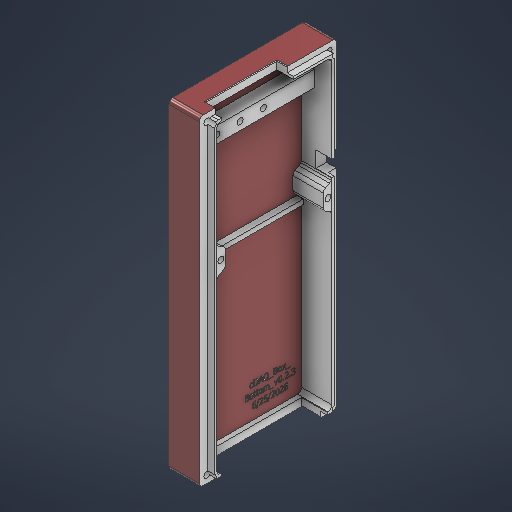
# Autodesk Inventor part: cDAQ_Box_Bottom_v0.2.3
Saved by Autodesk Inventor 2027 (Build 310192000, 192)
## iProperties
Created: 2026-05-08
Part Number: cDAQ_Box_Bottom_v0.2.3
Material: Generic
Document SubType Name: Modeling
Designer: giese
Density: 1 g/cm^3
Appearance: Default
Author: giese
Autodesk Inventor part; units mm, degrees
(part 1 of 2)
ref_plane "YZ Plane" through (0, 0, 0) normal (1, 0, 0) x (0, 1, 0)
ref_plane "XZ Plane" through (0, 0, 0) normal (0, 1, 0) x (-1, 0, 0)
ref_plane "XY Plane" through (0, 0, 0) normal (0, 0, 1) x (1, 0, 0)
sketch "Sketch1" plane through (0, 0, 0) normal (1, 0, 0) x (0, 1, 0)
  line L0 (37.5698, 60.7867) -> (-217.4462, 60.7867)
  line L1 (-217.4462, 60.7867) -> (-217.4462, -48.4333)
  line L2 (-217.4462, -48.4333) -> (37.5698, -48.4333)
  line L3 (37.5698, -48.4333) -> (37.5698, 60.7867)
  point P0 (0, 0)
  dimension "d0" = 109.22
  dimension "d1" = 255.016
  constraints: 8 end point, 2 parallel, 1 horizontal, 1 perpendicular
  measures "d0" distance of L2.end L0.start
  measures "d1" distance of L1.end L2.end
extrude "Extrusion1" add sketch "Sketch1" along normal blind 24.13
sketch "Sketch2" plane through (24.13, 0, 0) normal (1, 0, 0) x (0, 0, -1)
  line L0 (39.5433, 31.2198) -> (-51.8967, 31.2198)
  line L1 (-51.8967, 31.2198) -> (-51.8967, -211.0962)
  line L2 (-51.8967, -211.0962) -> (39.5433, -211.0962)
  line L3 (39.5433, -211.0962) -> (39.5433, 31.2198)
  line L4 (48.4333, 37.5698) -> (-60.7867, 37.5698) projected
  line L5 (-60.7867, 37.5698) -> (-60.7867, -217.4462) projected
  line L6 (-60.7867, -217.4462) -> (48.4333, -217.4462) projected
  line L7 (48.4333, -217.4462) -> (48.4333, 37.5698) projected
  point P0 (0, 0)
  dimension "d4" = 242.316
  dimension "d5" = 91.44
  dimension "d8" = 6.35
  dimension "d21" = 8.89
  dimension "d690" = 6.35
  dimension "d842" = 8.89
  constraints: 8 end point, 2 parallel, 1 horizontal, 1 perpendicular
  measures "d4" distance of L2.end L0.start
  measures "d5" distance of L0.start L0.end
  measures "d8" distance between parallel lines of L0 L4
  measures "d21" distance between parallel lines of L5 L1
  measures "d690" distance between parallel lines of L6 L2
  measures "d842" distance between parallel lines of L7 L3
extrude "Extrusion2" cut sketch "Sketch2" against normal blind 19.05 contours L3 L2 L1 L0
sketch "Sketch3" plane through (0, 0, 0) normal (-1, 0, 0) x (0, 0, 1)
  circle A0 centre (0.9291, 9.6298) radius 2.4005
  circle A1 centre (19.4279, 9.6298) radius 2.4005
  circle A2 centre (37.9267, 9.6298) radius 2.4005
  line L0 (-48.4333, -217.4462) -> (-48.4333, 37.5698) projected
  line L1 (-48.4333, 37.5698) -> (60.7867, 37.5698) projected
  line L2 (60.7867, 37.5698) -> (60.7867, -217.4462) projected
  line L3 (51.8967, 31.2198) -> (-39.5433, 31.2198) projected
  point P0 (0, 0)
  point P1 (-0.896, -23.7433)
  point P2 (-45.1848, 27.0137)
  dimension "d9" = 18.4988
  dimension "d10" = 4.801
  dimension "d11" = 4.801
  dimension "d12" = 18.4988
  dimension "d13" = 36.9976
  dimension "d18" = 22.86
  dimension "d22" = 4.801
  dimension "d58" = 27.94
  constraints: 3 centre point
  measures "d9" distance of A0.centre A1.centre
  measures "d10" diameter of A1
  measures "d11" diameter of A2
  measures "d12" distance of A1.centre A2.centre
  measures "d13" distance of A0.centre A2.centre
  measures "d18" distance from line of L2 A2.centre
  measures "d22" diameter of A0
  measures "d58" distance from line of L1 A2.centre
extrude "Extrusion3" cut sketch "Sketch3" against normal blind 5.08
sketch "Sketch5" plane through (0, -217.4462, -48.4333) normal (0, 0, -1) x (-1, 0, 0)
  line L0 (-27.2034, 165.862) -> (-16.51, 165.862)
  line L1 (-16.51, 165.862) -> (-16.51, 178.562)
  line L2 (-16.51, 178.562) -> (-27.2034, 178.562)
  line L3 (-27.2034, 178.562) -> (-27.2034, 165.862)
  line L4 (0, 255.016) -> (-24.13, 255.016) projected
  line L5 (0, 0) -> (0, 255.016) projected
  line L6 (-24.13, 0) -> (-24.13, 255.016) projected
  line L7 (0, 0) -> (-24.13, 0) projected
  point P0 (0, 217.4462)
  point P1 (-21.8567, 178.562)
  point P2 (-21.8567, 165.862)
  dimension "d28" = 10.6934
  dimension "d30" = 12.7
  dimension "d31" = 16.51
  dimension "d215" = 3.0734
  dimension "d1133" = 165.862
  constraints: 8 end point, 2 midpoint, 2 parallel, 1 horizontal, 1 perpendicular
  measures "d28" distance between parallel lines of L1 L3
  measures "d30" distance of point (-21.857, 178.562) point (-21.857, 165.862)
  measures "d31" distance between parallel lines of L5 L1
  measures "d215" distance between parallel lines of L6 L3
  measures "d1133" distance between parallel lines of L7 L0
extrude "Extrusion4" cut sketch "Sketch5" against normal blind 24.13 contours L3 L2 L6 L0 | L6 L2 L1 L0
sketch "Sketch6" plane through (0, -217.4462, -48.4333) normal (0, -1, 0) x (1, 0, 0)
  line L0 (24.08, 55.136) -> (16.08, 55.136)
  line L1 (16.08, 45.136) -> (24.08, 45.136)
  line L2 (0, 109.22) -> (0, 0) projected
  line L3 (29.63, 53.1359) -> (29.63, 47.136)
  line L4 (24.08, 55.136) -> (29.63, 53.1359)
  line L5 (29.63, 47.136) -> (24.08, 45.136)
  line L6 (0, 0) -> (24.13, 0) projected
  line L7 (24.13, 100.33) -> (24.13, 8.89) projected
  line L8 (24.13, 41.9134) -> (24.13, 37.4697)
  line L9 (16.08, 55.136) -> (8.636, 55.136)
  line L10 (8.636, 55.136) -> (8.636, 45.136)
  line L11 (8.636, 45.136) -> (21.16, 45.136)
  point P0 (0, 48.4333)
  point P1 (20.08, 55.136)
  point P2 (20.08, 45.136)
  point P3 (16.08, 50.136)
  dimension "d39" = 6
  dimension "d48" = 55.136
  dimension "d221" = 0
  dimension "d223" = 2
  dimension "d224" = 2
  dimension "d225" = 5.5
  dimension "d227" = 5.55
  dimension "d672" = 8.636
  constraints: 18 end point, 2 horizontal, 2 midpoint, 2 parallel, 2 point on line, 1 perpendicular, 1 vertical
  measures "d39" distance of L3.start L3.end
  measures "d48" distance between parallel lines of L6 L0
  measures "d221" horizontal distance of L0.start L1.end
  measures "d223" vertical distance of L3.end L1.end
  measures "d224" vertical distance of L0.start L3.start
  measures "d225" distance between parallel lines of L3 L7
  measures "d227" distance from line of L1.end L3
  measures "d672" distance between parallel lines of L2 L10
extrude "Extrusion5" [suppressed]
sketch "Sketch7" plane through (0, 37.5698, 60.7867) normal (0, 1, 0) x (1, 0, 0)
  line L0 (31.0134, 69.85) -> (16.002, 69.85)
  line L1 (16.002, 69.85) -> (16.002, 12.7)
  line L2 (16.002, 12.7) -> (31.0134, 12.7)
  line L3 (31.0134, 12.7) -> (31.0134, 69.85)
  line L4 (0, 0) -> (24.13, 0) projected
  line L5 (0, 109.22) -> (0, 0) projected
  line L6 (24.13, 109.22) -> (24.13, 0) projected
  point P0 (0, 60.7867)
  point P1 (24.13, 69.85)
  point P2 (24.13, 12.7)
  dimension "d52" = 12.7
  dimension "d55" = 16.002
  dimension "d56" = 15.0114
  dimension "d57" = 6.8834
  dimension "d1195" = 69.85
  constraints: 8 end point, 2 parallel, 1 horizontal, 1 perpendicular
  measures "d52" distance between parallel lines of L4 L2
  measures "d55" distance between parallel lines of L5 L1
  measures "d56" distance between parallel lines of L3 L1
  measures "d57" distance between parallel lines of L6 L3
  measures "d1195" distance between parallel lines of L4 L0
extrude "Extrusion6" cut sketch "Sketch7" against normal blind 7.62
fillet "Fillet1" radius 3.175 4 edges at (12.065, 37.5698, -48.4333) (12.065, 37.5698, 60.7867) (12.065, -217.4462, -48.4333) (12.065, -217.4462, 60.7867)
sketch "Sketch8" plane through (0, 0, 0) normal (-1, 0, 0) x (0, 0, 1)
  line L0 (-0.8425, 6.0992) -> (2.6881, 6.0992)
  line L1 (-0.8425, 13.1604) -> (2.6881, 13.1604)
  line L2 (-0.8425, 6.0992) -> (-2.8809, 9.6298)
  line L3 (-0.8425, 13.1604) -> (-2.8809, 9.6298)
  line L4 (2.6881, 6.0992) -> (4.7264, 9.6298)
  line L5 (2.6881, 13.1604) -> (4.7264, 9.6298)
  circle A0 centre (0.9291, 9.6298) radius 2.4005 projected
  line L6 (17.6563, 6.0992) -> (21.1869, 6.0992)
  line L7 (17.6563, 13.1604) -> (21.1869, 13.1604)
  line L8 (17.6563, 6.0992) -> (15.6179, 9.6298)
  line L9 (17.6563, 13.1604) -> (15.6179, 9.6298)
  line L10 (21.1869, 6.0992) -> (23.2253, 9.6298)
  line L11 (21.1869, 13.1604) -> (23.2253, 9.6298)
  circle A1 centre (19.4279, 9.6298) radius 2.4005 projected
  line L12 (36.1551, 6.0992) -> (34.1167, 9.6298)
  line L13 (36.1551, 13.1604) -> (34.1167, 9.6298)
  line L14 (36.1551, 6.0992) -> (39.6857, 6.0992)
  line L15 (36.1551, 13.1604) -> (39.6857, 13.1604)
  line L16 (39.6857, 6.0992) -> (41.7241, 9.6298)
  line L17 (39.6857, 13.1604) -> (41.7241, 9.6298)
  circle A2 centre (37.9267, 9.6298) radius 2.4005 projected
  point P0 (0.9228, 6.0992)
  point P1 (19.4216, 6.0992)
  point P2 (37.9204, 6.0992)
  point P3 (-2.8809, 9.6298)
  point P4 (4.7264, 9.6298)
  point P5 (23.2253, 9.6298)
  point P6 (15.6179, 9.6298)
  point P7 (41.7241, 9.6298)
  point P8 (34.1167, 9.6298)
  dimension "d60" = 7.0612
  dimension "d61" = 120
  dimension "d62" = 120
  dimension "d63" = 120
  dimension "d64" = 120
  dimension "d65" = 3.5306
  dimension "d66" = 3.5306
  dimension "d67" = 3.5306
  dimension "d68" = 3.5306
  dimension "d69" = 3.5306
  dimension "d70" = 3.5306
  dimension "d71" = 0
  dimension "d72" = 7.6074
  dimension "d73" = 3.81
  dimension "d74" = 0
  dimension "d75" = 7.0612
  dimension "d76" = 120
  dimension "d77" = 120
  dimension "d78" = 120
  dimension "d79" = 120
  dimension "d80" = 3.5306
  dimension "d81" = 3.5306
  dimension "d82" = 3.5306
  dimension "d83" = 3.5306
  dimension "d84" = 3.5306
  dimension "d85" = 3.5306
  dimension "d86" = 0
  dimension "d87" = 7.6074
  dimension "d91" = 0
  dimension "d92" = 3.81
  dimension "d93" = 7.0612
  dimension "d94" = 120
  dimension "d95" = 120
  dimension "d96" = 120
  dimension "d97" = 120
  dimension "d98" = 3.5306
  dimension "d99" = 3.5306
  dimension "d100" = 3.5306
  dimension "d101" = 3.5306
  dimension "d102" = 3.5306
  dimension "d103" = 3.5306
  dimension "d104" = 0
  dimension "d105" = 7.6074
  dimension "d108" = 0
  dimension "d109" = 3.81
  constraints: 36 end point, 6 horizontal, 3 midpoint
  measures "d60" distance from line of point (0.923, 6.099) L1
  measures "d61" angle of L0 L2
  measures "d62" angle of L1 L3
  measures "d63" angle of L4 L0
  measures "d64" angle of L5 L1
  measures "d65" distance of L0.start L0.end
  measures "d66" distance of L1.start L1.end
  measures "d67" vertical distance of L1.start L3.end
  measures "d68" vertical distance of L0.start L2.end
  measures "d69" vertical distance of L1.end L5.end
  measures "d70" vertical distance of L0.end L4.end
  measures "d71" horizontal distance of L0.start L1.start
  measures "d72" distance of L4.end L2.end
  measures "d73" distance of A0.centre L2.end
  measures "d74" vertical distance of A0.centre L4.end
  measures "d75" distance from line of point (19.422, 6.099) L7
  measures "d76" angle of L6 L8
  measures "d77" angle of L7 L9
  measures "d78" angle of L10 L6
  measures "d79" angle of L11 L7
  measures "d80" distance of L8.start L6.end
  measures "d81" distance of L9.start L7.end
  measures "d82" vertical distance of L9.start L9.end
  measures "d83" vertical distance of L8.start L8.end
  measures "d84" vertical distance of L7.end L11.end
  measures "d85" vertical distance of L6.end L10.end
  measures "d86" horizontal distance of L8.start L9.start
  measures "d87" distance of L10.end L8.end
  measures "d91" vertical distance of A1.centre L8.end
  measures "d92" distance of A1.centre L8.end
  measures "d93" distance from line of point (37.92, 6.099) L15
  measures "d94" angle of L14 L12
  measures "d95" angle of L15 L13
  measures "d96" angle of L16 L14
  measures "d97" angle of L17 L15
  measures "d98" distance of L12.start L16.start
  measures "d99" distance of L15.start L15.end
  measures "d100" vertical distance of L15.start L13.end
  measures "d101" vertical distance of L12.start L12.end
  measures "d102" vertical distance of L15.end L17.end
  measures "d103" vertical distance of L16.start L16.end
  measures "d104" horizontal distance of L12.start L15.start
  measures "d105" distance of L16.end L12.end
  measures "d108" vertical distance of A2.centre L12.end
  measures "d109" distance of A2.centre L12.end
extrude "Extrusion7" cut sketch "Sketch8" against normal blind 5 contours L2 L3 L1 L5 L4 L0 | A0 | L8 L9 L7 L11 L10 L6 | A1 | L12 L13 L15 L17 L16 L14 | A2
sketch "Sketch9" plane through (5.08, 0, 0) normal (1, 0, 0) x (0, 0, -1)
  arc A0 (22.2689, -180.8044) -> (16.8127, -180.8044) centre (19.5408, -178.3302) ccw
  line L0 (45.2583, 37.5698) -> (9.0633, 37.5698) projected
  line L1 (39.5433, 31.2198) -> (39.5433, -38.8842) projected
  arc A1 (17.6358, -185.9502) -> (21.4458, -185.9502) centre (19.5408, -185.9502) ccw
  line L2 (21.4458, -185.9502) -> (21.4458, -182.9374)
  line L3 (17.6358, -185.9502) -> (17.6358, -182.9374)
  arc A2 (22.2689, -180.8044) -> (21.4458, -182.9374) centre (24.6208, -182.9374) ccw
  arc A3 (17.6358, -182.9374) -> (16.8127, -180.8044) centre (14.4608, -182.9374) ccw
  arc A4 (-28.5311, -180.8044) -> (-33.9873, -180.8045) centre (-31.2592, -178.3302) ccw
  arc A5 (-33.1642, -185.9366) -> (-29.3542, -185.9502) centre (-31.2592, -185.9502) ccw
  line L4 (-29.3542, -185.9502) -> (-29.3542, -182.9374)
  line L5 (-33.1642, -185.9366) -> (-33.1642, -182.9374)
  arc A6 (-28.5311, -180.8044) -> (-29.3542, -182.9374) centre (-26.1792, -182.9374) ccw
  arc A7 (-33.1642, -182.9374) -> (-33.9873, -180.8045) centre (-36.3392, -182.9374) ccw
  line L6 (-48.0867, 37.5698) -> (-57.6117, 37.5698) projected
  line L7 (-51.8967, -211.0962) -> (-51.8967, 31.2198) projected
  point P0 (0, 0)
  point P1 (39.5433, -211.0962)
  point P2 (21.4458, -181.4823)
  point P3 (17.6358, -181.4823)
  point P4 (-29.3542, -181.4823)
  point P5 (-33.1642, -181.4823)
  point P6 (-51.8967, 31.2198)
  point P7 (-49.3567, -207.2862)
  dimension "d112" = 215.9
  dimension "d114" = 7.366
  dimension "d116" = 3.81
  dimension "d117" = 223.52
  dimension "d118" = 3.175
  dimension "d119" = 7.366
  dimension "d120" = 3.81
  dimension "d121" = 3.175
  dimension "d122" = 215.9
  dimension "d123" = 223.52
  dimension "d125" = 0
  dimension "d128" = 50.8
  dimension "d129" = 20.0025
  dimension "d130" = 0
  constraints: 20 point on circle, 8 centre point, 8 end point, 8 tangent, 4 point on line, 2 equal radius, 2 parallel, 2 vertical, 1 other
  measures "d112" distance from line of L0 A0.centre
  measures "d114" diameter of A0
  measures "d116" diameter of A1
  measures "d117" distance from line of L0 A1.centre
  measures "d118" radius of A2
  measures "d119" diameter of A4
  measures "d120" diameter of A5
  measures "d121" radius of A6
  measures "d122" distance from line of A4.centre L6
  measures "d123" distance from line of L6 A5.centre
  measures "d125" horizontal distance of A5.centre A4.centre
  measures "d128" distance of A5.centre A1.centre
  measures "d129" distance from line of L1 A0.centre
  measures "d130" horizontal distance of A0.centre A1.centre
extrude "Extrusion8" [suppressed]
sketch "Sketch10" plane through (24.13, 0, 0) normal (1, 0, 0) x (0, 0, -1)
  line L0 (-51.8967, 31.2198) -> (39.5433, 31.2198) projected
  line L1 (-51.8967, 31.2198) -> (39.5433, 31.2198)
  line L2 (42.0833, 33.2264) -> (-46.8167, 33.2264)
  line L3 (-46.8167, 33.2264) -> (-53.9033, 33.2264)
  line L4 (-53.9033, 33.2264) -> (-53.9033, -213.1028)
  line L5 (-53.9033, -213.1028) -> (41.5499, -213.1028)
  line L6 (41.5499, -213.1028) -> (41.5499, 33.2264)
  line L7 (41.5499, 33.2264) -> (41.9392, 33.2264)
  line L8 (39.5433, 31.2198) -> (39.5433, -38.8842) projected
  line L9 (-51.8967, -211.0962) -> (-51.8967, 31.2198) projected
  line L10 (39.5433, -211.0962) -> (-51.8967, -211.0962) projected
  line L11 (45.2583, 37.5698) -> (9.0633, 37.5698) projected
  line L12 (39.5433, 31.2198) -> (39.5433, -211.0962)
  line L13 (39.5433, -211.0962) -> (-51.8967, -211.0962)
  line L14 (-57.6117, -217.4462) -> (45.2583, -217.4462) projected
  line L15 (-51.8967, -211.0962) -> (-51.8967, 31.2198)
  line L16 (-51.8967, 31.2198) -> (39.5433, 31.2198)
  line L17 (-51.8967, 31.2198) -> (39.5433, 31.2198)
  line L18 (39.5433, 31.2198) -> (39.5433, -211.0962)
  line L19 (39.5433, -211.0962) -> (-51.8967, -211.0962)
  line L20 (-51.8967, -211.0962) -> (-51.8967, 31.2198)
  point P0 (41.5499, 33.2264)
  point P1 (-49.3567, -207.2862)
  point P2 (39.5433, -38.8842)
  dimension "d202" = 2.0066
  dimension "d203" = 2.0066
  dimension "d204" = 2.0066
  dimension "d205" = 2.0066
  dimension "d208" = 4.3434
  constraints: 30 end point, 6 perpendicular, 3 collinear, 3 point on line, 2 horizontal, 2 parallel, 2 other
  measures "d202" distance between parallel lines of L0 L2
  measures "d203" distance between parallel lines of L6 L8
  measures "d205" distance between parallel lines of L5 L10
  measures "d208" distance between parallel lines of L11 L2
extrude "Extrusion9" add sketch "Sketch10" along normal blind 5
fillet "Fillet2" radius 3.175 7 edges at (17.105, 31.2198, -39.5433) (17.105, 31.2198, 51.8967) (17.105, -211.0962, 51.8967) (17.105, -211.0962, -39.5433) (26.63, 33.2264, 53.9033) (26.63, -213.1028, -41.5499) (26.63, -213.1028, 53.9033)
sketch "Sketch13" plane through (29.13, 0, 0) normal (1, 0, 0) x (0, 0, -1)
  arc A0 (44.0833, 30.0448) -> (40.9083, 33.2198) centre (40.9083, 30.0448) ccw projected
  arc A1 (-45.6417, 33.2198) -> (-48.8167, 30.0448) centre (-45.6417, 30.0448) ccw projected
  arc A2 (40.9083, -212.0802) -> (44.0833, -208.9052) centre (40.9083, -208.9052) ccw projected
  arc A3 (-48.8167, -208.9052) -> (-45.6417, -212.0802) centre (-45.6417, -208.9052) ccw projected
  line L0 (-48.0867, 37.5698) -> (-57.6117, 37.5698) projected
  line L1 (-60.7867, 34.3948) -> (-60.7867, -214.2712) projected
  line L2 (-57.6117, -217.4462) -> (45.2583, -217.4462) projected
  arc A4 (-48.8167, -208.9052) -> (-45.6417, -212.0802) centre (-45.6417, -208.9052) ccw projected
  circle A5 centre (-54.6907, -211.3502) radius 2.4005
  circle A6 centre (42.3373, -211.3502) radius 2.4005
  line L3 (48.4333, -214.2712) -> (48.4333, 34.3948) projected
  circle A7 centre (42.3373, 31.4738) radius 2.4005
  line L4 (45.2583, 37.5698) -> (9.0633, 37.5698) projected
  circle A8 centre (-54.6907, 31.4738) radius 2.4005
  arc A9 (41.4904, -28.6131) -> (38.3154, -25.4381) centre (38.3154, -28.6131) ccw
  circle A10 centre (36.3683, -64.0302) radius 2.4005
  circle A11 centre (-48.7217, -64.0302) radius 2.4005
  point P0 (0, 0)
  point P1 (-47.8868, 32.2898)
  point P2 (-47.8868, -211.1503)
  point P3 (-47.8868, -211.1503)
  point P4 (45.8404, -24.2631)
  point P5 (42.6654, -21.0881)
  dimension "d178" = 6.096
  dimension "d179" = 6.096
  dimension "d180" = 4.801
  dimension "d181" = 6.096
  dimension "d182" = 6.096
  dimension "d183" = 4.801
  dimension "d184" = 4.801
  dimension "d185" = 6.096
  dimension "d186" = 6.096
  dimension "d187" = 4.801
  dimension "d188" = 6.096
  dimension "d189" = 6.096
  dimension "d326" = 4.801
  dimension "d327" = 12.065
  dimension "d328" = 101.6
  dimension "d329" = 4.801
  dimension "d330" = 12.065
  dimension "d331" = 101.6
  constraints: 7 centre point, 5 point on circle
  measures "d178" distance from line of L1 A5.centre
  measures "d179" distance from line of L2 A5.centre
  measures "d180" diameter of A5
  measures "d181" distance from line of L2 A6.centre
  measures "d182" distance from line of L3 A6.centre
  measures "d183" diameter of A6
  measures "d184" diameter of A7
  measures "d185" distance from line of L3 A7.centre
  measures "d186" distance from line of L4 A7.centre
  measures "d187" diameter of A8
  measures "d188" distance from line of L0 A8.centre
  measures "d189" distance from line of L1 A8.centre
  measures "d326" diameter of A10
  measures "d327" distance from line of L3 A10.centre
  measures "d328" distance from line of A10.centre L4
  measures "d329" diameter of A11
  measures "d330" distance from line of L1 A11.centre
  measures "d331" distance from line of L0 A11.centre
extrude "Extrusion11" cut sketch "Sketch13" against normal blind 25.4
sketch "Sketch14" plane through (5.08, 0, 0) normal (1, 0, 0) x (0, 0, -1)
  line L0 (4.9426, -183.8597) -> (24.1593, -183.8597) construction
  line L1 (24.1593, -183.8597) -> (24.1593, -181.9103) construction
  line L2 (24.1593, -181.9103) -> (4.9426, -181.9103) construction
  line L3 (4.9426, -181.9103) -> (4.9426, -183.8597) construction
  spline S0 degree 2 poles (0.0458, -188.6059) (-0.3099, -188.6059) (-0.899, -188.3873) (-1.1102, -188.165) knots 0 0 0 1 2 2 2
  spline S1 degree 2 poles (-1.1102, -188.165) (-1.3214, -187.9464) (-1.5548, -187.2721) (-1.5548, -186.82) knots 0 0 0 1 2 2 2
  spline S2 degree 2 poles (-1.5548, -186.82) (-1.5548, -186.368) (-1.314, -185.7085) (-1.1102, -185.4862) knots 0 0 0 1 2 2 2
  spline S3 degree 2 poles (-1.1102, -185.4862) (-0.9064, -185.2602) (-0.3025, -185.0194) (0.0458, -185.0194) knots 0 0 0 1 2 2 2
  spline S4 degree 2 poles (0.0458, -185.0194) (0.3273, -185.0194) (0.8535, -185.1787) (1.0572, -185.2825) knots 0 0 0 1 2 2 2
  line L4 (1.0572, -185.2825) -> (1.0572, -185.9308)
  line L5 (1.0572, -185.9308) -> (1.0239, -185.9308)
  spline S5 degree 2 poles (1.0239, -185.9308) (0.9609, -185.879) (0.7682, -185.7456) (0.6312, -185.6752) knots 0 0 0 1 2 2 2
  spline S6 degree 2 poles (0.6312, -185.6752) (0.5089, -185.6159) (0.1829, -185.5233) (0.0347, -185.5233) knots 0 0 0 1 2 2 2
  spline S7 degree 2 poles (0.0347, -185.5233) (-0.4137, -185.5233) (-0.9583, -186.2013) (-0.9583, -186.82) knots 0 0 0 1 2 2 2
  spline S8 degree 2 poles (-0.9583, -186.82) (-0.9583, -187.424) (-0.4322, -188.102) (0.0347, -188.102) knots 0 0 0 1 2 2 2
  spline S9 degree 2 poles (0.0347, -188.102) (0.3162, -188.102) (0.8275, -187.8686) (1.0239, -187.687) knots 0 0 0 1 2 2 2
  line L6 (1.0239, -187.687) -> (1.0572, -187.687)
  line L7 (1.0572, -187.687) -> (1.0572, -188.3354)
  spline S10 degree 2 poles (1.0572, -188.3354) (0.972, -188.3762) (0.7127, -188.491) (0.6089, -188.5169) knots 0 0 0 1 2 2 2
  spline S11 degree 2 poles (0.6089, -188.5169) (0.4607, -188.5614) (0.2273, -188.6059) (0.0458, -188.6059) knots 0 0 0 1 2 2 2
  spline S12 degree 2 poles (5.2328, -186.2458) (5.2328, -186.8719) (4.7252, -187.8797) (4.2991, -188.1613) knots 0 0 0 1 2 2 2
  spline S13 degree 2 poles (4.2991, -188.1613) (3.9509, -188.3799) (3.2358, -188.5281) (2.68, -188.5281) knots 0 0 0 1 2 2 2
  line L8 (2.68, -188.5281) -> (1.6278, -188.5281)
  line L9 (1.6278, -188.5281) -> (1.6278, -183.9561)
  line L10 (1.6278, -183.9561) -> (2.6689, -183.9561)
  spline S14 degree 2 poles (2.6689, -183.9561) (3.3136, -183.9561) (4.0472, -184.1487) (4.3065, -184.3191) knots 0 0 0 1 2 2 2
  spline S15 degree 2 poles (4.3065, -184.3191) (4.7474, -184.6118) (5.2328, -185.5789) (5.2328, -186.2458) knots 0 0 0 1 2 2 2
  spline S16 degree 2 poles (4.5992, -186.2384) (4.5992, -185.7122) (4.251, -184.9675) (3.9064, -184.7563) knots 0 0 0 1 2 2 2
  spline S17 degree 2 poles (3.9064, -184.7563) (3.6619, -184.6118) (3.1098, -184.4822) (2.6986, -184.4822) knots 0 0 0 1 2 2 2
  line L11 (2.6986, -184.4822) -> (2.2354, -184.4822)
  line L12 (2.2354, -184.4822) -> (2.2354, -188.0019)
  line L13 (2.2354, -188.0019) -> (2.6986, -188.0019)
  spline S18 degree 2 poles (2.6986, -188.0019) (3.1024, -188.0019) (3.7137, -187.8723) (3.962, -187.6981) knots 0 0 0 1 2 2 2
  spline S19 degree 2 poles (3.962, -187.6981) (4.2806, -187.4832) (4.5992, -186.7719) (4.5992, -186.2384) knots 0 0 0 1 2 2 2
  line L14 (5.3995, -188.5281) -> (6.9408, -183.9561)
  line L15 (6.9408, -183.9561) -> (7.6892, -183.9561)
  line L16 (7.6892, -183.9561) -> (9.2305, -188.5281)
  line L17 (9.2305, -188.5281) -> (8.5896, -188.5281)
  line L18 (8.5896, -188.5281) -> (8.1746, -187.2498)
  line L19 (8.1746, -187.2498) -> (6.4295, -187.2498)
  line L20 (6.4295, -187.2498) -> (6.0146, -188.5281)
  line L21 (6.0146, -188.5281) -> (5.3995, -188.5281)
  line L22 (8.0079, -186.7311) -> (7.3002, -184.5785)
  line L23 (7.3002, -184.5785) -> (6.5962, -186.7311)
  line L24 (6.5962, -186.7311) -> (8.0079, -186.7311)
  spline S20 degree 2 poles (13.4617, -189.647) (13.2949, -189.6877) (12.9318, -189.7322) (12.7503, -189.7322) knots 0 0 0 1 2 2 2
  spline S21 degree 2 poles (12.7503, -189.7322) (12.2353, -189.7322) (11.5943, -189.1579) (11.5647, -188.6244) knots 0 0 0 1 2 2 2
  spline S22 degree 2 poles (11.5647, -188.6244) (11.5239, -188.6244) (11.4535, -188.6244) (11.4239, -188.6244) knots 0 0 0 1 2 2 2
  spline S23 degree 2 poles (11.4239, -188.6244) (10.9608, -188.6244) (10.2161, -188.3095) (9.9493, -188.0019) knots 0 0 0 1 2 2 2
  spline S24 degree 2 poles (9.9493, -188.0019) (9.6862, -187.6981) (9.4047, -186.8089) (9.4047, -186.2458) knots 0 0 0 1 2 2 2
  spline S25 degree 2 poles (9.4047, -186.2458) (9.4047, -185.6678) (9.6899, -184.7934) (9.953, -184.4822) knots 0 0 0 1 2 2 2
  spline S26 degree 2 poles (9.953, -184.4822) (10.2198, -184.1747) (10.9645, -183.8597) (11.4239, -183.8597) knots 0 0 0 1 2 2 2
  spline S27 degree 2 poles (11.4239, -183.8597) (11.8907, -183.8597) (12.6391, -184.1858) (12.8985, -184.4822) knots 0 0 0 1 2 2 2
  spline S28 degree 2 poles (12.8985, -184.4822) (13.1578, -184.7823) (13.4468, -185.6752) (13.4468, -186.2458) knots 0 0 0 1 2 2 2
  spline S29 degree 2 poles (13.4468, -186.2458) (13.4468, -187.135) (12.754, -188.2909) (12.1501, -188.4947) knots 0 0 0 1 2 2 2
  spline S30 degree 2 poles (12.1501, -188.4947) (12.1649, -188.6651) (12.2538, -188.9393) (12.3242, -189.0171) knots 0 0 0 1 2 2 2
  spline S31 degree 2 poles (12.3242, -189.0171) (12.4094, -189.1135) (12.6428, -189.2024) (12.8503, -189.2024) knots 0 0 0 1 2 2 2
  spline S32 degree 2 poles (12.8503, -189.2024) (12.9726, -189.2024) (13.306, -189.1246) (13.3801, -189.0949) knots 0 0 0 1 2 2 2
  line L25 (13.3801, -189.0949) -> (13.4617, -189.0949)
  line L26 (13.4617, -189.0949) -> (13.4617, -189.647)
  spline S33 degree 2 poles (12.8133, -186.2458) (12.8133, -185.79) (12.6169, -185.0898) (12.4391, -184.8601) knots 0 0 0 1 2 2 2
  spline S34 degree 2 poles (12.4391, -184.8601) (12.2575, -184.623) (11.7462, -184.3858) (11.4276, -184.3858) knots 0 0 0 1 2 2 2
  spline S35 degree 2 poles (11.4276, -184.3858) (11.0979, -184.3858) (10.6014, -184.6156) (10.4124, -184.8601) knots 0 0 0 1 2 2 2
  spline S36 degree 2 poles (10.4124, -184.8601) (10.2309, -185.0935) (10.0382, -185.8012) (10.0382, -186.2458) knots 0 0 0 1 2 2 2
  spline S37 degree 2 poles (10.0382, -186.2458) (10.0382, -187.1461) (10.794, -188.1057) (11.4276, -188.1057) knots 0 0 0 1 2 2 2
  spline S38 degree 2 poles (11.4276, -188.1057) (12.0612, -188.1057) (12.8133, -187.1461) (12.8133, -186.2458) knots 0 0 0 1 2 2 2
  line L27 (17.1296, -189.4469) -> (13.6024, -189.4469)
  line L28 (13.6024, -189.4469) -> (13.6024, -189.0505)
  line L29 (13.6024, -189.0505) -> (17.1296, -189.0505)
  line L30 (17.1296, -189.0505) -> (17.1296, -189.4469)
  spline S39 degree 2 poles (20.6457, -187.1239) (20.6457, -187.4647) (20.3863, -187.9871) (20.1715, -188.1576) knots 0 0 0 1 2 2 2
  spline S40 degree 2 poles (20.1715, -188.1576) (19.9121, -188.3576) (19.323, -188.5281) (18.8562, -188.5281) knots 0 0 0 1 2 2 2
  line L31 (18.8562, -188.5281) -> (17.5446, -188.5281)
  line L32 (17.5446, -188.5281) -> (17.5446, -183.9561)
  line L33 (17.5446, -183.9561) -> (18.7561, -183.9561)
  spline S41 degree 2 poles (18.7561, -183.9561) (19.2452, -183.9561) (19.7343, -184.019) (19.9566, -184.1413) knots 0 0 0 1 2 2 2
  spline S42 degree 2 poles (19.9566, -184.1413) (20.2048, -184.271) (20.4308, -184.6971) (20.4308, -184.9861) knots 0 0 0 1 2 2 2
  spline S43 degree 2 poles (20.4308, -184.9861) (20.4308, -185.3084) (20.0899, -185.8197) (19.7898, -185.9642) knots 0 0 0 1 2 2 2
  line L34 (19.7898, -185.9642) -> (19.7898, -185.9864)
  spline S44 degree 2 poles (19.7898, -185.9864) (20.1974, -186.0976) (20.6457, -186.6867) (20.6457, -187.1239) knots 0 0 0 1 2 2 2
  spline S45 degree 2 poles (20.0121, -187.1498) (20.0121, -186.8904) (19.8639, -186.557) (19.6416, -186.4384) knots 0 0 0 1 2 2 2
  spline S46 degree 2 poles (19.6416, -186.4384) (19.4971, -186.3643) (19.1563, -186.3199) (18.8414, -186.3199) knots 0 0 0 1 2 2 2
  line L35 (18.8414, -186.3199) -> (18.1522, -186.3199)
  line L36 (18.1522, -186.3199) -> (18.1522, -188.0094)
  line L37 (18.1522, -188.0094) -> (18.645, -188.0094)
  spline S47 degree 2 poles (18.645, -188.0094) (19.0451, -188.0094) (19.5046, -187.9353) (19.6824, -187.8167) knots 0 0 0 1 2 2 2
  spline S48 degree 2 poles (19.6824, -187.8167) (19.8528, -187.6944) (20.0121, -187.3906) (20.0121, -187.1498) knots 0 0 0 1 2 2 2
  spline S49 degree 2 poles (19.7973, -185.0713) (19.7973, -184.9082) (19.6861, -184.6637) (19.5638, -184.5933) knots 0 0 0 1 2 2 2
  spline S50 degree 2 poles (19.5638, -184.5933) (19.4156, -184.5118) (19.0562, -184.4748) (18.7339, -184.4748) knots 0 0 0 1 2 2 2
  line L38 (18.7339, -184.4748) -> (18.1522, -184.4748)
  line L39 (18.1522, -184.4748) -> (18.1522, -185.8123)
  line L40 (18.1522, -185.8123) -> (18.8414, -185.8123)
  spline S51 degree 2 poles (18.8414, -185.8123) (19.1266, -185.8123) (19.3971, -185.753) (19.5416, -185.6604) knots 0 0 0 1 2 2 2
  spline S52 degree 2 poles (19.5416, -185.6604) (19.6824, -185.5714) (19.7973, -185.2862) (19.7973, -185.0713) knots 0 0 0 1 2 2 2
  spline S53 degree 2 poles (24.0247, -186.8126) (24.0247, -187.6796) (23.1911, -188.6244) (22.4945, -188.6244) knots 0 0 0 1 2 2 2
  spline S54 degree 2 poles (22.4945, -188.6244) (21.7794, -188.6244) (20.9606, -187.65) (20.9606, -186.8126) knots 0 0 0 1 2 2 2
  spline S55 degree 2 poles (20.9606, -186.8126) (20.9606, -185.9531) (21.8054, -185.0009) (22.4945, -185.0009) knots 0 0 0 1 2 2 2
  spline S56 degree 2 poles (22.4945, -185.0009) (23.1911, -185.0009) (24.0247, -185.9494) (24.0247, -186.8126) knots 0 0 0 1 2 2 2
  spline S57 degree 2 poles (23.4282, -186.8126) (23.4282, -186.1457) (22.9428, -185.4973) (22.4945, -185.4973) knots 0 0 0 1 2 2 2
  spline S58 degree 2 poles (22.4945, -185.4973) (22.0462, -185.4973) (21.5571, -186.1457) (21.5571, -186.8126) knots 0 0 0 1 2 2 2
  spline S59 degree 2 poles (21.5571, -186.8126) (21.5571, -187.461) (22.0462, -188.1279) (22.4945, -188.1279) knots 0 0 0 1 2 2 2
  spline S60 degree 2 poles (22.4945, -188.1279) (22.9391, -188.1279) (23.4282, -187.4721) (23.4282, -186.8126) knots 0 0 0 1 2 2 2
  line L41 (27.2814, -188.5281) -> (26.5737, -188.5281)
  line L42 (26.5737, -188.5281) -> (25.7401, -187.2387)
  line L43 (25.7401, -187.2387) -> (24.8842, -188.5281)
  line L44 (24.8842, -188.5281) -> (24.2285, -188.5281)
  line L45 (24.2285, -188.5281) -> (25.4178, -186.8275)
  line L46 (25.4178, -186.8275) -> (24.2396, -185.0972)
  line L47 (24.2396, -185.0972) -> (24.9472, -185.0972)
  line L48 (24.9472, -185.0972) -> (25.7772, -186.3754)
  line L49 (25.7772, -186.3754) -> (26.6256, -185.0972)
  line L50 (26.6256, -185.0972) -> (27.2814, -185.0972)
  line L51 (27.2814, -185.0972) -> (26.0995, -186.7904)
  line L52 (26.0995, -186.7904) -> (27.2814, -188.5281)
  line L53 (30.7901, -189.4469) -> (27.2629, -189.4469)
  line L54 (27.2629, -189.4469) -> (27.2629, -189.0505)
  line L55 (27.2629, -189.0505) -> (30.7901, -189.0505)
  line L56 (30.7901, -189.0505) -> (30.7901, -189.4469)
  spline S61 degree 2 poles (-2.2254, -194.6515) (-2.2254, -194.9924) (-2.4848, -195.5148) (-2.6997, -195.6852) knots 0 0 0 1 2 2 2
  spline S62 degree 2 poles (-2.6997, -195.6852) (-2.959, -195.8853) (-3.5481, -196.0557) (-4.0149, -196.0557) knots 0 0 0 1 2 2 2
  line L57 (-4.0149, -196.0557) -> (-5.3265, -196.0557)
  line L58 (-5.3265, -196.0557) -> (-5.3265, -191.4837)
  line L59 (-5.3265, -191.4837) -> (-4.115, -191.4837)
  spline S63 degree 2 poles (-4.115, -191.4837) (-3.6259, -191.4837) (-3.1369, -191.5467) (-2.9145, -191.669) knots 0 0 0 1 2 2 2
  spline S64 degree 2 poles (-2.9145, -191.669) (-2.6663, -191.7987) (-2.4403, -192.2247) (-2.4403, -192.5137) knots 0 0 0 1 2 2 2
  spline S65 degree 2 poles (-2.4403, -192.5137) (-2.4403, -192.8361) (-2.7812, -193.3474) (-3.0813, -193.4919) knots 0 0 0 1 2 2 2
  line L60 (-3.0813, -193.4919) -> (-3.0813, -193.5141)
  spline S66 degree 2 poles (-3.0813, -193.5141) (-2.6737, -193.6252) (-2.2254, -194.2143) (-2.2254, -194.6515) knots 0 0 0 1 2 2 2
  spline S67 degree 2 poles (-2.859, -194.6775) (-2.859, -194.4181) (-3.0072, -194.0847) (-3.2295, -193.9661) knots 0 0 0 1 2 2 2
  spline S68 degree 2 poles (-3.2295, -193.9661) (-3.374, -193.892) (-3.7148, -193.8475) (-4.0298, -193.8475) knots 0 0 0 1 2 2 2
  line L61 (-4.0298, -193.8475) -> (-4.7189, -193.8475)
  line L62 (-4.7189, -193.8475) -> (-4.7189, -195.537)
  line L63 (-4.7189, -195.537) -> (-4.2261, -195.537)
  spline S69 degree 2 poles (-4.2261, -195.537) (-3.826, -195.537) (-3.3666, -195.4629) (-3.1887, -195.3444) knots 0 0 0 1 2 2 2
  spline S70 degree 2 poles (-3.1887, -195.3444) (-3.0183, -195.2221) (-2.859, -194.9183) (-2.859, -194.6775) knots 0 0 0 1 2 2 2
  spline S71 degree 2 poles (-3.0739, -192.5989) (-3.0739, -192.4359) (-3.185, -192.1914) (-3.3073, -192.121) knots 0 0 0 1 2 2 2
  spline S72 degree 2 poles (-3.3073, -192.121) (-3.4555, -192.0395) (-3.8149, -192.0024) (-4.1372, -192.0024) knots 0 0 0 1 2 2 2
  line L64 (-4.1372, -192.0024) -> (-4.7189, -192.0024)
  line L65 (-4.7189, -192.0024) -> (-4.7189, -193.34)
  line L66 (-4.7189, -193.34) -> (-4.0298, -193.34)
  spline S73 degree 2 poles (-4.0298, -193.34) (-3.7445, -193.34) (-3.474, -193.2807) (-3.3295, -193.188) knots 0 0 0 1 2 2 2
  spline S74 degree 2 poles (-3.3295, -193.188) (-3.1887, -193.0991) (-3.0739, -192.8138) (-3.0739, -192.5989) knots 0 0 0 1 2 2 2
  spline S75 degree 2 poles (1.1536, -194.3403) (1.1536, -195.2073) (0.3199, -196.1521) (-0.3766, -196.1521) knots 0 0 0 1 2 2 2
  spline S76 degree 2 poles (-0.3766, -196.1521) (-1.0917, -196.1521) (-1.9105, -195.1776) (-1.9105, -194.3403) knots 0 0 0 1 2 2 2
  spline S77 degree 2 poles (-1.9105, -194.3403) (-1.9105, -193.4807) (-1.0657, -192.5286) (-0.3766, -192.5286) knots 0 0 0 1 2 2 2
  spline S78 degree 2 poles (-0.3766, -192.5286) (0.3199, -192.5286) (1.1536, -193.477) (1.1536, -194.3403) knots 0 0 0 1 2 2 2
  spline S79 degree 2 poles (0.5571, -194.3403) (0.5571, -193.6734) (0.0717, -193.025) (-0.3766, -193.025) knots 0 0 0 1 2 2 2
  spline S80 degree 2 poles (-0.3766, -193.025) (-0.8249, -193.025) (-1.314, -193.6734) (-1.314, -194.3403) knots 0 0 0 1 2 2 2
  spline S81 degree 2 poles (-1.314, -194.3403) (-1.314, -194.9887) (-0.8249, -195.6556) (-0.3766, -195.6556) knots 0 0 0 1 2 2 2
  spline S82 degree 2 poles (-0.3766, -195.6556) (0.068, -195.6556) (0.5571, -194.9998) (0.5571, -194.3403) knots 0 0 0 1 2 2 2
  spline S83 degree 2 poles (2.7838, -196.1224) (2.3132, -196.1224) (1.7834, -195.5852) (1.7834, -195.0035) knots 0 0 0 1 2 2 2
  line L67 (1.7834, -195.0035) -> (1.7834, -193.1028)
  line L68 (1.7834, -193.1028) -> (1.3944, -193.1028)
  line L69 (1.3944, -193.1028) -> (1.3944, -192.6249)
  line L70 (1.3944, -192.6249) -> (1.7834, -192.6249)
  line L71 (1.7834, -192.6249) -> (1.7834, -191.6393)
  line L72 (1.7834, -191.6393) -> (2.3614, -191.6393)
  line L73 (2.3614, -191.6393) -> (2.3614, -192.6249)
  line L74 (2.3614, -192.6249) -> (3.4247, -192.6249)
  line L75 (3.4247, -192.6249) -> (3.4247, -193.1028)
  line L76 (3.4247, -193.1028) -> (2.3614, -193.1028)
  line L77 (2.3614, -193.1028) -> (2.3614, -194.7367)
  spline S84 degree 2 poles (2.3614, -194.7367) (2.3614, -194.9961) (2.3799, -195.2814) (2.4429, -195.4036) knots 0 0 0 1 2 2 2
  spline S85 degree 2 poles (2.4429, -195.4036) (2.4948, -195.5111) (2.7282, -195.6185) (2.9283, -195.6185) knots 0 0 0 1 2 2 2
  spline S86 degree 2 poles (2.9283, -195.6185) (3.0691, -195.6185) (3.3321, -195.5333) (3.3914, -195.5074) knots 0 0 0 1 2 2 2
  line L78 (3.3914, -195.5074) -> (3.4247, -195.5074)
  line L79 (3.4247, -195.5074) -> (3.4247, -196.0261)
  spline S87 degree 2 poles (3.4247, -196.0261) (3.2617, -196.0706) (2.9283, -196.1224) (2.7838, -196.1224) knots 0 0 0 1 2 2 2
  spline S88 degree 2 poles (4.8882, -196.1224) (4.4177, -196.1224) (3.8879, -195.5852) (3.8879, -195.0035) knots 0 0 0 1 2 2 2
  line L80 (3.8879, -195.0035) -> (3.8879, -193.1028)
  line L81 (3.8879, -193.1028) -> (3.4988, -193.1028)
  line L82 (3.4988, -193.1028) -> (3.4988, -192.6249)
  line L83 (3.4988, -192.6249) -> (3.8879, -192.6249)
  line L84 (3.8879, -192.6249) -> (3.8879, -191.6393)
  line L85 (3.8879, -191.6393) -> (4.4659, -191.6393)
  line L86 (4.4659, -191.6393) -> (4.4659, -192.6249)
  line L87 (4.4659, -192.6249) -> (5.5292, -192.6249)
  line L88 (5.5292, -192.6249) -> (5.5292, -193.1028)
  line L89 (5.5292, -193.1028) -> (4.4659, -193.1028)
  line L90 (4.4659, -193.1028) -> (4.4659, -194.7367)
  spline S89 degree 2 poles (4.4659, -194.7367) (4.4659, -194.9961) (4.4844, -195.2814) (4.5474, -195.4036) knots 0 0 0 1 2 2 2
  spline S90 degree 2 poles (4.5474, -195.4036) (4.5992, -195.5111) (4.8327, -195.6185) (5.0327, -195.6185) knots 0 0 0 1 2 2 2
  spline S91 degree 2 poles (5.0327, -195.6185) (5.1735, -195.6185) (5.4366, -195.5333) (5.4959, -195.5074) knots 0 0 0 1 2 2 2
  line L91 (5.4959, -195.5074) -> (5.5292, -195.5074)
  line L92 (5.5292, -195.5074) -> (5.5292, -196.0261)
  spline S92 degree 2 poles (5.5292, -196.0261) (5.3662, -196.0706) (5.0327, -196.1224) (4.8882, -196.1224) knots 0 0 0 1 2 2 2
  spline S93 degree 2 poles (8.7748, -194.3403) (8.7748, -195.2073) (7.9412, -196.1521) (7.2446, -196.1521) knots 0 0 0 1 2 2 2
  spline S94 degree 2 poles (7.2446, -196.1521) (6.5296, -196.1521) (5.7107, -195.1776) (5.7107, -194.3403) knots 0 0 0 1 2 2 2
  spline S95 degree 2 poles (5.7107, -194.3403) (5.7107, -193.4807) (6.5555, -192.5286) (7.2446, -192.5286) knots 0 0 0 1 2 2 2
  spline S96 degree 2 poles (7.2446, -192.5286) (7.9412, -192.5286) (8.7748, -193.477) (8.7748, -194.3403) knots 0 0 0 1 2 2 2
  spline S97 degree 2 poles (8.1783, -194.3403) (8.1783, -193.6734) (7.6929, -193.025) (7.2446, -193.025) knots 0 0 0 1 2 2 2
  spline S98 degree 2 poles (7.2446, -193.025) (6.7963, -193.025) (6.3073, -193.6734) (6.3073, -194.3403) knots 0 0 0 1 2 2 2
  spline S99 degree 2 poles (6.3073, -194.3403) (6.3073, -194.9887) (6.7963, -195.6556) (7.2446, -195.6556) knots 0 0 0 1 2 2 2
  spline S100 degree 2 poles (7.2446, -195.6556) (7.6892, -195.6556) (8.1783, -194.9998) (8.1783, -194.3403) knots 0 0 0 1 2 2 2
  line L93 (13.2579, -196.0557) -> (13.2579, -194.0698)
  spline S101 degree 2 poles (13.2579, -194.0698) (13.2579, -193.8327) (13.2208, -193.4289) (13.1616, -193.3177) knots 0 0 0 1 2 2 2
  spline S102 degree 2 poles (13.1616, -193.3177) (13.1023, -193.1955) (12.8763, -193.0769) (12.6799, -193.0769) knots 0 0 0 1 2 2 2
  spline S103 degree 2 poles (12.6799, -193.0769) (12.5021, -193.0769) (12.0945, -193.2955) (11.8796, -193.503) knots 0 0 0 1 2 2 2
  spline S104 degree 2 poles (11.8796, -193.503) (11.8833, -193.5548) (11.8907, -193.6993) (11.8907, -193.7957) knots 0 0 0 1 2 2 2
  line L94 (11.8907, -193.7957) -> (11.8907, -196.0557)
  line L95 (11.8907, -196.0557) -> (11.3127, -196.0557)
  line L96 (11.3127, -196.0557) -> (11.3127, -194.0698)
  spline S105 degree 2 poles (11.3127, -194.0698) (11.3127, -193.8327) (11.2757, -193.4289) (11.2164, -193.3177) knots 0 0 0 1 2 2 2
  spline S106 degree 2 poles (11.2164, -193.3177) (11.1571, -193.1955) (10.9311, -193.0769) (10.7348, -193.0769) knots 0 0 0 1 2 2 2
  spline S107 degree 2 poles (10.7348, -193.0769) (10.5495, -193.0769) (10.1383, -193.3103) (9.9456, -193.4919) knots 0 0 0 1 2 2 2
  line L97 (9.9456, -193.4919) -> (9.9456, -196.0557)
  line L98 (9.9456, -196.0557) -> (9.3676, -196.0557)
  line L99 (9.3676, -196.0557) -> (9.3676, -192.6249)
  line L100 (9.3676, -192.6249) -> (9.9456, -192.6249)
  line L101 (9.9456, -192.6249) -> (9.9456, -193.0028)
  spline S108 degree 2 poles (9.9456, -193.0028) (10.1716, -192.7768) (10.6162, -192.5286) (10.883, -192.5286) knots 0 0 0 1 2 2 2
  spline S109 degree 2 poles (10.883, -192.5286) (11.1868, -192.5286) (11.6573, -192.8064) (11.7796, -193.1214) knots 0 0 0 1 2 2 2
  spline S110 degree 2 poles (11.7796, -193.1214) (12.0426, -192.8287) (12.5391, -192.5286) (12.8281, -192.5286) knots 0 0 0 1 2 2 2
  spline S111 degree 2 poles (12.8281, -192.5286) (13.0504, -192.5286) (13.4135, -192.6656) (13.5469, -192.8212) knots 0 0 0 1 2 2 2
  spline S112 degree 2 poles (13.5469, -192.8212) (13.684, -192.9769) (13.8359, -193.4437) (13.8359, -193.7957) knots 0 0 0 1 2 2 2
  line L102 (13.8359, -193.7957) -> (13.8359, -196.0557)
  line L103 (13.8359, -196.0557) -> (13.2579, -196.0557)
  line L104 (17.7076, -196.9746) -> (14.1804, -196.9746)
  line L105 (14.1804, -196.9746) -> (14.1804, -196.5781)
  line L106 (14.1804, -196.5781) -> (17.7076, -196.5781)
  line L107 (17.7076, -196.5781) -> (17.7076, -196.9746)
  line L108 (20.7717, -192.6249) -> (19.4786, -196.0557)
  line L109 (19.4786, -196.0557) -> (18.9599, -196.0557)
  line L110 (18.9599, -196.0557) -> (17.678, -192.6249)
  line L111 (17.678, -192.6249) -> (18.3041, -192.6249)
  line L112 (18.3041, -192.6249) -> (19.2415, -195.2666)
  line L113 (19.2415, -195.2666) -> (20.1715, -192.6249)
  line L114 (20.1715, -192.6249) -> (20.7717, -192.6249)
  spline S113 degree 2 poles (23.9691, -193.7697) (23.9691, -194.9998) (23.254, -196.1521) (22.5093, -196.1521) knots 0 0 0 1 2 2 2
  spline S114 degree 2 poles (22.5093, -196.1521) (21.7535, -196.1521) (21.0458, -194.9776) (21.0458, -193.7734) knots 0 0 0 1 2 2 2
  spline S115 degree 2 poles (21.0458, -193.7734) (21.0458, -192.536) (21.7609, -191.3911) (22.5093, -191.3911) knots 0 0 0 1 2 2 2
  spline S116 degree 2 poles (22.5093, -191.3911) (23.2614, -191.3911) (23.9691, -192.5767) (23.9691, -193.7697) knots 0 0 0 1 2 2 2
  spline S117 degree 2 poles (23.1836, -195.1628) (23.2726, -194.9368) (23.3467, -194.2403) (23.3467, -193.7697) knots 0 0 0 1 2 2 2
  spline S118 degree 2 poles (23.3467, -193.7697) (23.3467, -193.2992) (23.2726, -192.6064) (23.1799, -192.3729) knots 0 0 0 1 2 2 2
  spline S119 degree 2 poles (23.1799, -192.3729) (23.0873, -192.1395) (22.765, -191.8987) (22.5093, -191.8987) knots 0 0 0 1 2 2 2
  spline S120 degree 2 poles (22.5093, -191.8987) (22.2537, -191.8987) (21.9239, -192.1395) (21.8276, -192.3804) knots 0 0 0 1 2 2 2
  spline S121 degree 2 poles (21.8276, -192.3804) (21.735, -192.6138) (21.6683, -193.3251) (21.6683, -193.7734) knots 0 0 0 1 2 2 2
  spline S122 degree 2 poles (21.6683, -193.7734) (21.6683, -194.2551) (21.7276, -194.8998) (21.8239, -195.1517) knots 0 0 0 1 2 2 2
  spline S123 degree 2 poles (21.8239, -195.1517) (21.9128, -195.3888) (22.2426, -195.6445) (22.5093, -195.6445) knots 0 0 0 1 2 2 2
  spline S124 degree 2 poles (22.5093, -195.6445) (22.7613, -195.6445) (23.091, -195.4036) (23.1836, -195.1628) knots 0 0 0 1 2 2 2
  line L115 (25.5363, -196.0557) -> (24.8027, -196.0557)
  line L116 (24.8027, -196.0557) -> (24.8027, -195.1813)
  line L117 (24.8027, -195.1813) -> (25.5363, -195.1813)
  line L118 (25.5363, -195.1813) -> (25.5363, -196.0557)
  line L119 (29.2784, -196.0557) -> (26.4589, -196.0557)
  line L120 (26.4589, -196.0557) -> (26.4589, -195.4074)
  spline S125 degree 2 poles (26.4589, -195.4074) (26.7627, -195.1221) (27.3036, -194.5922) (27.563, -194.307) knots 0 0 0 1 2 2 2
  spline S126 degree 2 poles (27.563, -194.307) (28.0854, -193.7327) (28.467, -193.0435) (28.467, -192.6768) knots 0 0 0 1 2 2 2
  spline S127 degree 2 poles (28.467, -192.6768) (28.467, -192.4841) (28.3484, -192.1951) (28.241, -192.1025) knots 0 0 0 1 2 2 2
  spline S128 degree 2 poles (28.241, -192.1025) (28.1336, -192.0098) (27.852, -191.9172) (27.6815, -191.9172) knots 0 0 0 1 2 2 2
  spline S129 degree 2 poles (27.6815, -191.9172) (27.5185, -191.9172) (27.1851, -191.9987) (27.0332, -192.0617) knots 0 0 0 1 2 2 2
  spline S130 degree 2 poles (27.0332, -192.0617) (26.9035, -192.1136) (26.6627, -192.2618) (26.5886, -192.3137) knots 0 0 0 1 2 2 2
  line L121 (26.5886, -192.3137) -> (26.5552, -192.3137)
  line L122 (26.5552, -192.3137) -> (26.5552, -191.6616)
  spline S131 degree 2 poles (26.5552, -191.6616) (26.7442, -191.5689) (27.4222, -191.3874) (27.726, -191.3874) knots 0 0 0 1 2 2 2
  spline S132 degree 2 poles (27.726, -191.3874) (28.367, -191.3874) (29.0895, -192.0654) (29.0895, -192.6434) knots 0 0 0 1 2 2 2
  spline S133 degree 2 poles (29.0895, -192.6434) (29.0895, -192.9139) (28.9635, -193.3659) (28.8523, -193.5585) knots 0 0 0 1 2 2 2
  spline S134 degree 2 poles (28.8523, -193.5585) (28.7412, -193.7586) (28.4188, -194.1514) (28.241, -194.3403) knots 0 0 0 1 2 2 2
  spline S135 degree 2 poles (28.241, -194.3403) (27.952, -194.6552) (27.2443, -195.3295) (27.0332, -195.5259) knots 0 0 0 1 2 2 2
  line L123 (27.0332, -195.5259) -> (29.2784, -195.5259)
  line L124 (29.2784, -195.5259) -> (29.2784, -196.0557)
  line L125 (30.8716, -196.0557) -> (30.138, -196.0557)
  line L126 (30.138, -196.0557) -> (30.138, -195.1813)
  line L127 (30.138, -195.1813) -> (30.8716, -195.1813)
  line L128 (30.8716, -195.1813) -> (30.8716, -196.0557)
  spline S136 degree 2 poles (33.0279, -191.9172) (32.8612, -191.9172) (32.5314, -191.9987) (32.3721, -192.0617) knots 0 0 0 1 2 2 2
  spline S137 degree 2 poles (32.3721, -192.0617) (32.2239, -192.1247) (32.0053, -192.2581) (31.9201, -192.3174) knots 0 0 0 1 2 2 2
  line L129 (31.9201, -192.3174) -> (31.883, -192.3174)
  line L130 (31.883, -192.3174) -> (31.883, -191.669)
  spline S138 degree 2 poles (31.883, -191.669) (32.0831, -191.5615) (32.7685, -191.3874) (33.0761, -191.3874) knots 0 0 0 1 2 2 2
  spline S139 degree 2 poles (33.0761, -191.3874) (33.3873, -191.3874) (33.8504, -191.5134) (34.0394, -191.6468) knots 0 0 0 1 2 2 2
  spline S140 degree 2 poles (34.0394, -191.6468) (34.2394, -191.7913) (34.4469, -192.2099) (34.4469, -192.4915) knots 0 0 0 1 2 2 2
  spline S141 degree 2 poles (34.4469, -192.4915) (34.4469, -192.8694) (33.9504, -193.44) (33.6022, -193.5141) knots 0 0 0 1 2 2 2
  line L131 (33.6022, -193.5141) -> (33.6022, -193.5585)
  spline S142 degree 2 poles (33.6022, -193.5585) (33.7467, -193.5882) (34.0764, -193.7216) (34.2172, -193.8549) knots 0 0 0 1 2 2 2
  spline S143 degree 2 poles (34.2172, -193.8549) (34.358, -193.9846) (34.5358, -194.3996) (34.5358, -194.6997) knots 0 0 0 1 2 2 2
  spline S144 degree 2 poles (34.5358, -194.6997) (34.5358, -195.0072) (34.3246, -195.5296) (34.132, -195.7297) knots 0 0 0 1 2 2 2
  spline S145 degree 2 poles (34.132, -195.7297) (33.9319, -195.9372) (33.365, -196.1521) (33.0057, -196.1521) knots 0 0 0 1 2 2 2
  spline S146 degree 2 poles (33.0057, -196.1521) (32.6611, -196.1521) (31.9868, -195.9853) (31.7571, -195.8705) knots 0 0 0 1 2 2 2
  line L132 (31.7571, -195.8705) -> (31.7571, -195.2221)
  line L133 (31.7571, -195.2221) -> (31.8015, -195.2221)
  spline S147 degree 2 poles (31.8015, -195.2221) (31.9942, -195.3629) (32.6463, -195.6222) (32.9686, -195.6222) knots 0 0 0 1 2 2 2
  spline S148 degree 2 poles (32.9686, -195.6222) (33.1576, -195.6222) (33.5355, -195.5037) (33.6615, -195.3666) knots 0 0 0 1 2 2 2
  spline S149 degree 2 poles (33.6615, -195.3666) (33.7837, -195.2295) (33.9134, -194.9035) (33.9134, -194.6552) knots 0 0 0 1 2 2 2
  spline S150 degree 2 poles (33.9134, -194.6552) (33.9134, -194.407) (33.7689, -194.0847) (33.6392, -193.992) knots 0 0 0 1 2 2 2
  spline S151 degree 2 poles (33.6392, -193.992) (33.5095, -193.8994) (33.1576, -193.829) (32.9501, -193.829) knots 0 0 0 1 2 2 2
  line L134 (32.9501, -193.829) -> (32.6907, -193.829)
  line L135 (32.6907, -193.829) -> (32.6907, -193.3214)
  line L136 (32.6907, -193.3214) -> (32.8945, -193.3214)
  spline S152 degree 2 poles (32.8945, -193.3214) (33.3058, -193.3214) (33.8245, -192.9287) (33.8245, -192.5545) knots 0 0 0 1 2 2 2
  spline S153 degree 2 poles (33.8245, -192.5545) (33.8245, -192.3804) (33.6911, -192.1321) (33.5836, -192.058) knots 0 0 0 1 2 2 2
  spline S154 degree 2 poles (33.5836, -192.058) (33.4688, -191.9802) (33.1872, -191.9172) (33.0279, -191.9172) knots 0 0 0 1 2 2 2
  spline S155 degree 2 poles (3.3618, -202.1014) (3.3618, -202.4534) (3.1283, -203.0499) (2.932, -203.25) knots 0 0 0 1 2 2 2
  spline S156 degree 2 poles (2.932, -203.25) (2.7282, -203.4611) (2.2169, -203.6797) (1.9094, -203.6797) knots 0 0 0 1 2 2 2
  spline S157 degree 2 poles (1.9094, -203.6797) (1.6019, -203.6797) (1.0943, -203.4723) (0.9016, -203.2648) knots 0 0 0 1 2 2 2
  spline S158 degree 2 poles (0.9016, -203.2648) (0.6645, -203.0165) (0.3977, -202.1829) (0.3977, -201.5753) knots 0 0 0 1 2 2 2
  spline S159 degree 2 poles (0.3977, -201.5753) (0.3977, -200.9788) (0.6423, -200.0192) (0.8979, -199.6635) knots 0 0 0 1 2 2 2
  spline S160 degree 2 poles (0.8979, -199.6635) (1.1462, -199.3152) (1.9316, -198.9262) (2.4466, -198.9262) knots 0 0 0 1 2 2 2
  spline S161 degree 2 poles (2.4466, -198.9262) (2.5985, -198.9262) (2.8653, -198.9558) (2.9653, -198.9892) knots 0 0 0 1 2 2 2
  line L137 (2.9653, -198.9892) -> (2.9653, -199.5783)
  line L138 (2.9653, -199.5783) -> (2.9394, -199.5783)
  spline S162 degree 2 poles (2.9394, -199.5783) (2.8542, -199.5338) (2.543, -199.456) (2.3651, -199.456) knots 0 0 0 1 2 2 2
  spline S163 degree 2 poles (2.3651, -199.456) (1.7945, -199.456) (1.0943, -200.2267) (1.0276, -200.9825) knots 0 0 0 1 2 2 2
  spline S164 degree 2 poles (1.0276, -200.9825) (1.2462, -200.8306) (1.7056, -200.6639) (1.9798, -200.6639) knots 0 0 0 1 2 2 2
  spline S165 degree 2 poles (1.9798, -200.6639) (2.2466, -200.6639) (2.6467, -200.7713) (2.8653, -200.9343) knots 0 0 0 1 2 2 2
  spline S166 degree 2 poles (2.8653, -200.9343) (3.1172, -201.1233) (3.3618, -201.7087) (3.3618, -202.1014) knots 0 0 0 1 2 2 2
  spline S167 degree 2 poles (2.7393, -202.1273) (2.7393, -201.8458) (2.5911, -201.4641) (2.4281, -201.3308) knots 0 0 0 1 2 2 2
  spline S168 degree 2 poles (2.4281, -201.3308) (2.3058, -201.2344) (2.002, -201.1714) (1.8427, -201.1714) knots 0 0 0 1 2 2 2
  spline S169 degree 2 poles (1.8427, -201.1714) (1.6278, -201.1714) (1.224, -201.3011) (1.0276, -201.4234) knots 0 0 0 1 2 2 2
  spline S170 degree 2 poles (1.0276, -201.4234) (1.0239, -201.4901) (1.0165, -201.616) (1.0165, -201.7124) knots 0 0 0 1 2 2 2
  spline S171 degree 2 poles (1.0165, -201.7124) (1.0165, -202.1866) (1.2017, -202.7683) (1.3425, -202.9202) knots 0 0 0 1 2 2 2